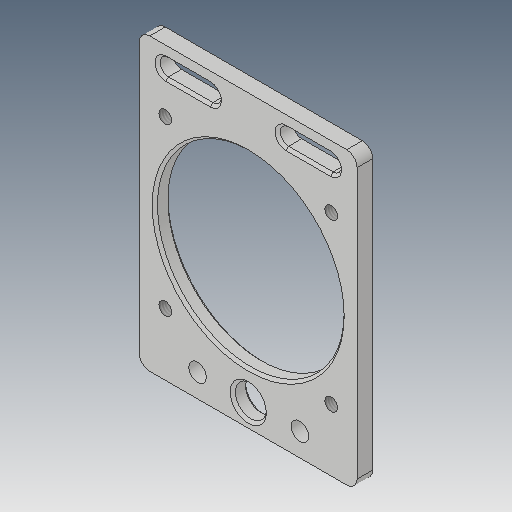
# Autodesk Inventor part: fan bracket
Saved by Autodesk Inventor 2019 (Build 230136000, 136)
## iProperties
Created: 2018-11-13
Part Number: fan bracket
Material: Generic
Document SubType Name: Modeling
Designer: LillaHunden
Density: 1 g/cm^3
Appearance: Default
Mass: 3.53808 g
Surface Area: 35.8898 cm^2
Volume: 3.53808 cm^3
Author: LillaHunden
Autodesk Inventor part; units mm, degrees
ref_plane "YZ Plane" through (0, 0, 0) normal (1, 0, 0) x (0, 1, 0)
ref_plane "XZ Plane" through (0, 0, 0) normal (0, 1, 0) x (-1, 0, 0)
ref_plane "XY Plane" through (0, 0, 0) normal (0, 0, 1) x (1, 0, 0)
sketch "Sketch1" plane through (0, 0, 0) normal (0, 0, 1) x (1, 0, 0)
  line L0 (-21, -28) -> (21, -28)
  line L1 (21, -28) -> (21, 28)
  line L2 (21, 28) -> (-21, 28)
  line L3 (-21, 28) -> (-21, -28)
  line L4 (-21, -28) -> (21, 28) construction
  line L5 (21, -28) -> (-21, 28) construction
  point P0 (0, 0)
  dimension "d0" = 42
  dimension "d1" = 56
  constraints: 12 end point, 2 midpoint, 2 parallel, 1 horizontal, 1 perpendicular
  measures "d0" distance of L2.end L1.end
  measures "d1" distance of L1.end L0.end
extrude "Extrusion1" add sketch "Sketch1" along normal blind 3
sketch "Sketch2" plane through (0, 0, 3) normal (0, 0, 1) x (1, 0, 0)
  circle A0 centre (0, 0) radius 18
  dimension "d4" = 36
  constraints: 1 centre point, 1 coincident
  measures "d4" diameter of A0
extrude "Extrusion2" cut sketch "Sketch2" against normal through all
chamfer "Chamfer1" distance 0.5 angle 45 2 edges at (-18, 0, 3) (-18, 0, 0)
fillet "Fillet1" radius 2 4 edges at (21, 28, 1.5) (-21, 28, 1.5) (-21, -28, 1.5) (21, -28, 1.5)
sketch "Sketch3" plane through (0, 0, 3) normal (0, 0, 1) x (1, 0, 0)
  circle A0 centre (0, -23.7) radius 3
  line L0 (-2.3284, -26.7) -> (3.1329, -26.7)
  line L1 (-19, -28) -> (19, -28) projected
  point P0 (0, 0)
  dimension "d11" = 6
  dimension "d12" = 1.3
  constraints: 2 end point, 1 centre point, 1 parallel, 1 tangent
  measures "d11" diameter of A0
  measures "d12" distance between parallel lines of L1 L0
extrude "Extrusion3" cut sketch "Sketch3" against normal through all
chamfer "Chamfer2" distance 0.5 angle 45 2 edges at (-3, -23.7, 3) (-3, -23.7, 0)
sketch "Sketch4" plane through (0, 0, 3) normal (0, 0, 1) x (1, 0, 0)
  line L0 (-16, 16) -> (-16, -16) construction
  line L1 (-16, -16) -> (16, -16) construction
  point P0 (0, 0)
  point P1 (16, 16)
  point P2 (-16, 0)
  point P3 (0, -16)
  dimension "d18" = 32
  dimension "d19" = 32
  dimension "d20" = 32
  dimension "d21" = 32
  constraints: 4 end point, 2 midpoint, 1 horizontal, 1 horizontal alignment, 1 vertical, 1 vertical alignment
  measures "d18" distance of L1.end L0.end
  measures "d19" distance of point (16, 16) L1.end
  measures "d20" distance of L0.start L0.end
  measures "d21" distance of point (16, 16) L0.start
hole "Hole1" at (-16, 16, 3) at (16, 16, 3) at (16, -16, 3) at (-16, -16, 3) direction (0, 0, -1) diameter 2.459 depth 8.8 tip angle 118 thread size "M3x0.5" class "6H" standard "ISO Metric profile"
sketch "Sketch5" plane through (0, 0, 3) normal (0, 0, 1) x (1, 0, 0)
  line L0 (-17.5, 24.105) -> (-5.67, 24.105) construction
  line L1 (-15.875, 22.48) -> (-7.295, 22.48)
  line L2 (-7.295, 25.73) -> (-15.875, 25.73)
  arc A0 (-15.875, 25.73) -> (-15.875, 22.48) centre (-15.875, 24.105) ccw
  arc A1 (-7.295, 22.48) -> (-7.295, 25.73) centre (-7.295, 24.105) ccw
  line L3 (19, 28) -> (-19, 28) projected
  line L4 (-21, 26) -> (-21, -26) projected
  point P0 (0, 0)
  point P1 (-11.585, 24.105)
  dimension "d29" = 11.83
  dimension "d30" = 3.25
  dimension "d31" = 2.27
  dimension "d32" = 3.5
  constraints: 8 end point, 6 point on circle, 4 tangent, 2 centre point, 2 point on line, 1 horizontal, 1 midpoint, 1 parallel
  measures "d29" distance of L0.start L0.end
  measures "d30" diameter of A1
  measures "d31" distance between parallel lines of L3 L2
  measures "d32" distance from line of L4 L0.start
extrude "Extrusion4" cut sketch "Sketch5" against normal blind 3
ref_plane "Work Plane1" through (0, -26, 0) normal (-1, 0, 0) x (0, 0, 1)
mirror "Mirror1" about plane through (0, -26, 0) normal (-1, 0, 0) of "Extrusion4"
chamfer "Chamfer3" distance 0.5 angle 45 8 edges at (-11.585, 25.73, 3) (-5.67, 24.105, 3) (-11.585, 22.48, 3) (-17.5, 24.105, 3) (11.585, 25.73, 3) (17.5, 24.105, 3) (11.585, 22.48, 3) (5.67, 24.105, 3)
sketch "Sketch6" plane through (0, 0, 0) normal (0, 0, -1) x (-1, 0, 0)
  point P0 (-9.9708, -23.545)
hole "Hole2" at (9.9708, -23.545, 0) direction (0, 0, 1) diameter 3.4 depth 3
sketch "Sketch7" plane through (0, 0, 0) normal (0, 0, -1) x (-1, 0, 0)
  point P0 (9.7739, -23.545)
hole "Hole4" at (-9.7739, -23.545, 0) direction (0, 0, 1) diameter 3.4 depth 3
equation "\"d19\" = d18"
equation "\"d20\" = d18"
equation "\"d21\" = d18"
body "Solid1"
